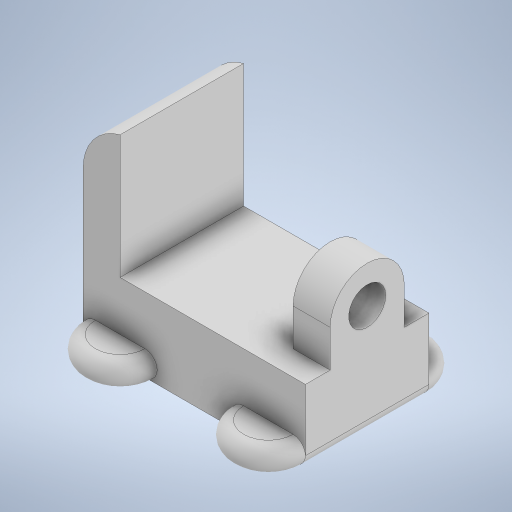
# Autodesk Inventor part: Lab 1B A
Saved by Autodesk Inventor 2024 (Build 280153000, 153)
## iProperties
Created: 2023-09-15
Part Number: Lab 1B A
Material: Generic
Document SubType Name: Modeling
Designer: furqa
Mass: 189.874 g
Surface Area: 285.259 cm^2
Volume: 189.874 cm^3
Density: 1 g/cm^3
Appearance: Default
Author: furqa
Autodesk Inventor part; units mm, degrees
ref_plane "YZ Plane" through (0, 0, 0) normal (1, 0, 0) x (0, 1, 0)
ref_plane "XZ Plane" through (0, 0, 0) normal (0, 1, 0) x (-1, 0, 0)
ref_plane "XY Plane" through (0, 0, 0) normal (0, 0, 1) x (1, 0, 0)
sketch "Sketch1" plane through (0, 0, 0) normal (0, 0, 1) x (1, 0, 0)
  line L0 (0, 0) -> (0, 60)
  line L1 (15, 80) -> (15, 30)
  line L2 (15, 30) -> (90, 30)
  line L3 (90, 30) -> (90, 0)
  line L4 (90, 0) -> (0, 0)
  arc A0 (15, 80) -> (0, 60) centre (19.99, 60.6325) ccw
  dimension "d0" = 60
  dimension "d1" = 90
  dimension "d2" = 30
  dimension "d3" = 75
  dimension "d4" = 50
  dimension "d5" = 20
  constraints: 10 end point, 3 perpendicular, 2 point on circle, 1 centre point, 1 vertical
  measures "d0" distance of L0.start L0.end
  measures "d1" distance of L3.end L0.start
  measures "d2" distance of L2.end L3.end
  measures "d3" distance from line of L2.end L1
  measures "d4" distance of L1.start L1.end
  measures "d5" radius of A0
extrude "Extrusion1" add sketch "Sketch1" along normal mid plane 50
sketch "Sketch2" plane through (90, 0, 25) normal (1, 0, 0) x (0, 0, -1)
  line L0 (50, 30) -> (0, 30) projected
  arc A0 (40, 45) -> (10, 45) centre (25, 45) ccw
  line L1 (50, 0) -> (0, 0) projected
  line L2 (50, 80) -> (50, 30) projected
  line L3 (10, 45) -> (10, 30)
  line L4 (40, 45) -> (40, 30)
  circle A1 centre (25, 45) radius 7.5
  point P0 (25, 0)
  dimension "d10" = 45
  dimension "d11" = 25
  dimension "d13" = 15
  dimension "d14" = 15
  constraints: 4 end point, 2 centre point, 2 perpendicular, 2 point on circle, 2 point on line, 1 coincident, 1 tangent
  measures "d10" distance from line of L1 A0.centre
  measures "d11" distance from line of L2 A0.centre
  measures "d13" radius of A0
  measures "d14" diameter of A1
extrude "Extrusion2" add sketch "Sketch2" against normal blind 15
sketch "Sketch3" plane through (0, 0, 25) normal (0, 0, 1) x (1, 0, 0)
  point P0 (0, 0)
sketch "Sketch5" plane through (0, 0, 25) normal (0, -1, 0) x (1, 0, 0)
  line L0 (90, 0) -> (15, 0) projected
  line L1 (0, 0) -> (90, 0) projected
  circle A0 centre (15, 0) radius 15
  circle A1 centre (75, 0) radius 15
  point P0 (0, -25)
  point P1 (60, 0)
  point P2 (30, 0)
  dimension "d18" = 30
  constraints: 1 point on line, 6 other
extrude "Extrusion3" add sketch "Sketch5" against normal blind 10 contours L0 L1 A0 | L0 A1 picked at (5.1453, 1.1966) picked at (70.6847, 5.6392)
full round fillet "Full Round Fillet2" first side at (70, 10, 31.6312) centre faces at (60.1942, 3.3333, 27.4062) second side at (50, 0, -8.3333)
sketch "Sketch7" plane through (0, 0, -25) normal (0, -1, 0) x (1, 0, 0)
  line L0 (15, 0) -> (90, 0) projected
  line L1 (90, 0) -> (0, 0) projected
  circle A0 centre (15, 0) radius 15
  circle A1 centre (75, 0) radius 15
  line L2 (0, 0) -> (0, 50) projected
  line L3 (90, 0) -> (90, 50) projected
  point P0 (0, 25)
  point P1 (30, 0)
  point P2 (60, 0)
  dimension "d21" = 30
  dimension "d22" = 30
  constraints: 2 point on line, 2 vertical, 6 other
extrude "Extrusion4" add sketch "Sketch7" against normal blind 10 contours L0 A0 L1 | L0 A1 picked at (24.8547, -1.1966) picked at (78.2678, -7.6351)
full round fillet "Full Round Fillet4" first side at (18.8878, 10, -29.5122) centre faces at (29.9514, 6.6667, -26.207) second side at (51.6666, 0, 8.3333)
fillet "Fillet1" radius 5 1 edges at (15, 10, 40)
fillet "Fillet2" radius 5 2 edges at (75, 10, -40) (75, 0, -40)
body "Solid1"
